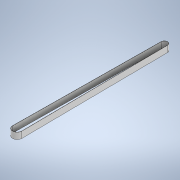
# Autodesk Inventor part: Belt
Saved by Autodesk Inventor 2020 (Build 240168000, 168)
## iProperties
Created: 2021-01-30
Part Number: Belt
Material: Generic
Document SubType Name: Modeling
Designer: kishore.balu
Density: 1 g/cm^3
Appearance: Default
Author: kishore.balu
Autodesk Inventor part; units mm, degrees
ref_plane "YZ Plane" through (0, 0, 0) normal (1, 0, 0) x (0, 1, 0)
ref_plane "XZ Plane" through (0, 0, 0) normal (0, 1, 0) x (-1, 0, 0)
ref_plane "XY Plane" through (0, 0, 0) normal (0, 0, 1) x (1, 0, 0)
sketch "Sketch1" plane through (0, 0, 0) normal (0, 1, 0) x (-1, 0, 0)
  arc A0 (5.9988, 187.329) -> (-5.9988, 187.329) centre (0, 187.45) ccw
  line L0 (6, 187.45) -> (4.1098, -0.0414)
  line L1 (-6, 187.45) -> (-4.11, 0)
  arc A1 (-3.86, 0.0012) -> (3.8598, -0.0389) centre (0, 0) ccw
  line L2 (-5.7488, 187.3328) -> (-5.75, 187.4525)
  arc A2 (5.7488, 187.3341) -> (-5.7488, 187.3341) centre (0, 187.45) ccw
  arc A3 (5.7488, 187.3328) -> (-5.7488, 187.3328) centre (0, 187.45) ccw
  arc A4 (-4.11, 0) -> (-3.8454, -1.451) centre (0, 0) ccw
  arc A5 (3.8456, -1.4504) -> (4.1098, -0.0414) centre (0, 0) ccw
  arc A6 (-4.11, 0) -> (4.1098, -0.0414) centre (0, 0) ccw
  line L3 (5.75, 187.4525) -> (5.7488, 187.3328)
  line L4 (5.7488, 187.3328) -> (3.8598, -0.0389)
  arc A7 (5.9988, 187.329) -> (-5.9988, 187.329) centre (0, 187.45) ccw
  line L5 (-5.75, 187.4525) -> (-5.7488, 187.3328)
  line L6 (-5.7488, 187.3328) -> (-3.86, 0.0012)
  point P0 (-5.75, 187.4512)
  point P1 (3.874, 1.3726)
  point P2 (5.7321, 185.6772)
  point P3 (-5.7321, 185.6772)
  point P4 (-3.8454, -1.451)
  point P5 (-5.7488, 187.3341)
  dimension "d1" = 12
  dimension "d4" = 0.25
  constraints: 18 point on circle, 14 end point, 8 centre point, 6 point on line, 3 coincident, 2 parallel, 1 concentric, 1 tangent
  measures "d1" diameter of A0
  measures "d4" radial gap between concentric circles of A0 A2
extrude "Extrusion1" add sketch "Sketch1" along normal blind 8
body "Solid1"
